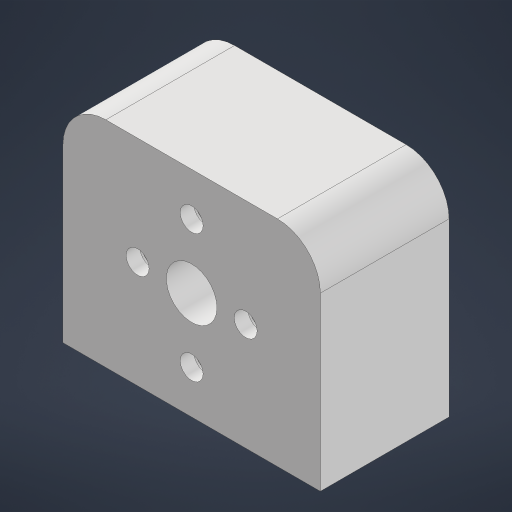
# Autodesk Inventor part: Motor Mounts
Saved by Autodesk Inventor 2023 (Build 270158000, 158)
## iProperties
Created: 2023-02-14
Part Number: Motor Mounts
Material: Generic
Document SubType Name: Modeling
Designer: Michael
Density: 1 g/cm^3
Appearance: Default
Author: Michael
Autodesk Inventor part; units mm, degrees
ref_plane "YZ Plane" through (0, 0, 0) normal (1, 0, 0) x (0, 1, 0)
ref_plane "XZ Plane" through (0, 0, 0) normal (0, 1, 0) x (-1, 0, 0)
ref_plane "XY Plane" through (0, 0, 0) normal (0, 0, 1) x (1, 0, 0)
sketch "Sketch1" plane through (0, 0, 0) normal (0, 0, 1) x (1, 0, 0)
  line L0 (0, 0) -> (38.1, 0)
  line L1 (38.1, 0) -> (38.1, 31.75)
  line L2 (38.1, 31.75) -> (0, 31.75)
  line L3 (0, 31.75) -> (0, 0)
  dimension "d0" = 38.1
  dimension "d1" = 31.75
  constraints: 8 end point, 2 parallel, 1 horizontal, 1 perpendicular
  measures "d0" distance of L2.end L1.end
  measures "d1" distance of L1.end L0.end
extrude "Extrusion1" add sketch "Sketch1" along normal blind 19.05
sketch "Sketch2" plane through (0, 0, 19.05) normal (0, 0, 1) x (1, 0, 0)
  line L0 (27.0485, 15.8754) -> (11.049, 15.8754)
  line L1 (19.0487, 6.3754) -> (19.0487, 25.3754)
  line L2 (0, 31.75) -> (0, 0)
  line L3 (38.1, 0) -> (0, 0)
  line L4 (0, 0) -> (38.1, 0) projected
  line L5 (0, 31.75) -> (0, 0) projected
  point P0 (19.0487, 15.8754)
  point P1 (0, -6.35)
  point P2 (9.525, -9.525)
  dimension "d4" = 15.9995
  dimension "d5" = 19
  dimension "d6" = 11.049
  dimension "d7" = 6.3754
  constraints: 6 end point, 4 coincident, 2 midpoint, 1 horizontal, 1 vertical, 3 other
  measures "d4" distance of L0.start L0.end
  measures "d5" distance of L1.start L1.end
  measures "d7" distance from line of L3 point (19.049, 6.375)
hole "Hole1" at (19.0487, 15.8754, 19.05) at (19.0487, 25.3754, 19.05) at (11.049, 15.8754, 19.05) at (19.0487, 6.3754, 19.05) at (27.0485, 15.8754, 19.05) direction (0, 0, -1) diameter 3.4036 depth 32.0675
sketch "Sketch3" plane through (0, 0, 0) normal (0, 0, -1) x (-1, 0, 0)
  circle A0 centre (-19.0487, 6.3754) radius 1.7018 projected
  circle A1 centre (-19.0487, 25.3754) radius 1.7018 projected
  circle A2 centre (-19.0487, 15.8754) radius 1.7018 projected
  circle A3 centre (-11.049, 15.8754) radius 1.7018 projected
  circle A4 centre (-27.0485, 15.8754) radius 1.7018 projected
  line L0 (-38.1, 0) -> (-38.1, 31.75) projected
  line L1 (0, 0) -> (-38.1, 0) projected
  line L2 (0, 31.75) -> (0, 0) projected
  line L3 (-38.1, 31.75) -> (0, 31.75) projected
  circle A5 centre (-19.0487, 25.3754) radius 1.7018 projected
  circle A6 centre (-19.0487, 6.3754) radius 1.7018 projected
  circle A7 centre (-19.0487, 15.8754) radius 1.7018 projected
  circle A8 centre (-19.0487, 15.8754) radius 5.5
  dimension "d34" = 11
  constraints: 6 coincident, 1 centre point
  measures "d34" diameter of A8
hole "Hole2" at (19.0487, 15.8754, 0) at (19.0487, 25.3754, 0) at (27.0485, 15.8754, 0) at (11.049, 15.8754, 0) at (19.0487, 6.3754, 0) direction (0, 0, 1) diameter 5.4356 depth 16.002
chamfer "Chamfer1" distance 1.016 angle 45 5 edges at (27.0485, 17.5772, 16.002) (19.0487, 27.0772, 16.002) (19.0487, 17.5772, 16.002) (11.049, 17.5772, 16.002) (19.0487, 8.0772, 16.002)
sketch "Sketch4" plane through (0, 0, 0) normal (0, -1, 0) x (1, 0, 0)
  line L0 (0, 0) -> (38.1, 0) projected
  line L1 (38.1, 0) -> (38.1, 19.05) projected
  line L2 (0, 19.05) -> (38.1, 19.05) projected
  line L3 (0, 0) -> (0, 19.05) projected
  line L4 (17.3469, 19.05) -> (20.7505, 19.05) projected
  line L5 (19.0487, 19.05) -> (19.05, 0)
  point P0 (8.128, 9.525)
  point P1 (29.9707, 9.5265)
  point P2 (0, 9.525)
  dimension "d25" = 9.525
  dimension "d26" = 8.128
  constraints: 3 midpoint, 2 end point, 1 symmetric about line
  measures "d25" distance from line of point (8.128, 9.525) L2
  measures "d26" distance of point (0, 9.525) point (8.128, 9.525)
hole "Hole3" at (8.128, 0, 9.525) at (29.9707, 0, 9.5265) direction (0, 1, 0) diameter 7.112 depth 10.414
sketch "Sketch5" plane through (0, 0, 19.05) normal (0, 0, 1) x (1, 0, 0)
  circle A0 centre (19.0487, 15.8754) radius 1.7018 projected
  circle A1 centre (19.0487, 15.8754) radius 3.75
  point P0 (0, 0)
  dimension "d35" = 7.5
  constraints: 1 centre point, 1 coincident
  measures "d35" diameter of A1
extrude "Extrusion2" cut sketch "Sketch5" against normal blind 25.4
fillet "Fillet2" radius 6.35 2 edges at (0, 31.75, 9.525) (38.1, 31.75, 9.525)
body "Solid1"
